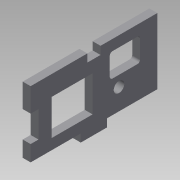
# Autodesk Inventor part: RJ45Plate
Saved by Autodesk Inventor 2013 (Build 170138000, 138)
## iProperties
Created: 2013-12-12
Part Number: RJ45Plate
Material: Generic
Document SubType Name: Modeling
Designer: Eric
Density: 1 g/cm^3
Author: Eric
Autodesk Inventor part; units mm, degrees
ref_plane "YZ Plane" through (0, 0, 0) normal (1, 0, 0) x (0, 1, 0)
ref_plane "XZ Plane" through (0, 0, 0) normal (0, 1, 0) x (-1, 0, 0)
ref_plane "XY Plane" through (0, 0, 0) normal (0, 0, 1) x (1, 0, 0)
sketch "Sketch1" plane through (0, 0, 0) normal (1, 0, 0) x (0, 1, 0)
  line L0 (18.5, 22.7485) -> (18.5, 25.7485)
  line L1 (23.5, 25.7485) -> (23.5, 22.7485)
  line L2 (0, 16.7485) -> (-3, 16.7485)
  line L3 (-3, 6.7485) -> (0, 6.7485)
  line L4 (16, 0.7485) -> (16, -2.2515)
  line L5 (16, -2.2515) -> (26, -2.2515)
  line L6 (26, -2.2515) -> (26, 0.7485)
  line L7 (26, 0.7485) -> (45, 0.7485)
  line L8 (23.5, 25.7485) -> (45, 25.7485)
  line L9 (18.5, 22.7485) -> (23.5, 22.7485)
  line L10 (-3, 16.7485) -> (-3, 25.7485)
  line L11 (-3, 6.7485) -> (-3, 0.7485)
  line L12 (-3, 25.7485) -> (18.5, 25.7485)
  line L13 (16, 0.7485) -> (-3, 0.7485)
  line L14 (45, 0.7485) -> (45, 25.7485)
  line L15 (0, 16.7485) -> (0, 6.7485)
  line L16 (5, 4.7485) -> (5, 18.2485)
  line L17 (5, 18.2485) -> (20.5, 18.2485)
  line L18 (20.5, 18.2485) -> (20.5, 4.7485)
  line L19 (20.5, 4.7485) -> (5, 4.7485)
  circle A0 centre (30.5, 8.7485) radius 2
  line L20 (27, 20.7485) -> (27, 13.7485)
  line L21 (28, 12.7485) -> (37.5, 12.7485)
  line L22 (38.5, 13.7485) -> (38.5, 20.7485)
  line L23 (37.5, 21.7485) -> (28, 21.7485)
  arc A1 (28, 21.7485) -> (27, 20.7485) centre (28, 20.7485) ccw
  arc A2 (38.5, 20.7485) -> (37.5, 21.7485) centre (37.5, 20.7485) ccw
  arc A3 (37.5, 12.7485) -> (38.5, 13.7485) centre (37.5, 13.7485) ccw
  arc A4 (27, 13.7485) -> (28, 12.7485) centre (28, 13.7485) ccw
  point P0 (27, 21.7485)
  point P1 (38.5, 12.7485)
  point P2 (27, 12.7485)
  dimension "d2" = 3
  dimension "d5" = 3
  dimension "d6" = 3
  dimension "d7" = 3
  dimension "d8" = 10
  dimension "d15" = 3
  dimension "d16" = 10
  dimension "d48" = 5
  dimension "d54" = 21.5
  dimension "d61" = 15.5
  dimension "d62" = 13.5
  dimension "d63" = 4
  dimension "d66" = 1
  dimension "d67" = 6.5
  dimension "d68" = 4
  dimension "d69" = 10
  dimension "d71" = 48
  dimension "d72" = 25
  dimension "d73" = 25
  dimension "d75" = 19
  dimension "d76" = 4
  dimension "d77" = 6.5
  dimension "d78" = 4
  dimension "d79" = 5
  dimension "d80" = 8
  dimension "d85" = 9
  constraints: 48 end point, 8 point on circle, 8 tangent, 7 parallel, 6 perpendicular, 6 point on line, 5 centre point, 3 equal radius, 1 collinear, 1 horizontal
  measures "d2" distance of L0.start L0.end
  measures "d5" distance of L1.start L1.end
  measures "d6" distance of L2.start L2.end
  measures "d7" distance of L3.start L3.end
  measures "d8" distance of L2.end L3.start
  measures "d15" distance of L4.start L4.end
  measures "d16" distance of L4.end L5.end
  measures "d48" distance between parallel lines of L1 L0
  measures "d54" distance between parallel lines of L10 L0
  measures "d61" distance of L17.start L18.start
  measures "d62" distance of L19.end L17.start
  measures "d63" diameter of A0
  measures "d66" radius of A1
  measures "d67" distance between parallel lines of L18 L20
  measures "d68" distance from line of A0.centre L21
  measures "d69" distance from line of L18 A0.centre
  measures "d71" distance between parallel lines of L10 L14
  measures "d72" distance between parallel lines of L7 L8
  measures "d73" distance between parallel lines of L13 L12
  measures "d75" distance of L4.start L11.end
  measures "d76" distance between parallel lines of L23 L8
  measures "d77" distance between parallel lines of L14 L22
  measures "d78" distance between parallel lines of L13 L19
  measures "d79" distance between parallel lines of L15 L16
  measures "d80" distance from line of L7 A0.centre
  measures "d85" distance of L2.end L10.end
extrude "Extrusion5" add sketch "Sketch1" along normal blind 3
body "Solid2"
